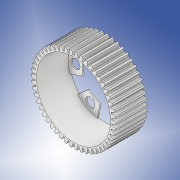
# Autodesk Inventor part: Flexspline
Saved by Autodesk Inventor 2017 SP1 (Build 210196100, 196)
## iProperties
Created: 2017-07-11
Part Number: Flexspline
Material: ABS Plastic
Document SubType Name: Modeling
Designer: zallen
Density: 1.06 g/cm^3
Appearance: CR White
Author: zallen
Autodesk Inventor part; units mm, degrees
ref_plane "YZ Plane" through (0, 0, 0) normal (1, 0, 0) x (0, 1, 0)
ref_plane "XZ Plane" through (0, 0, 0) normal (0, 1, 0) x (-1, 0, 0)
ref_plane "XY Plane" through (0, 0, 0) normal (0, 0, 1) x (1, 0, 0)
sketch "Sketch1" plane through (0, 0, 0) normal (0, 0, 1) x (1, 0, 0)
  circle A0 centre (0, 0) radius 29
  circle A1 centre (0, 0) radius 32 construction
  line L0 (0, 0) -> (52.2063, 0) construction
  arc A2 (31.9944, 0.6) -> (28.9662, 1.4) centre (26.6699, -13.4232) ccw
  arc A3 (31.9944, -0.6) -> (31.9944, 0.6) centre (12.0034, 0) ccw
  arc A4 (28.9662, -1.4) -> (31.9944, -0.6) centre (26.6699, 13.4232) ccw
  arc A5 (28.9662, -1.4) -> (28.9662, 1.4) centre (0, 0) ccw
  arc A6 (31.6669, 4.6052) -> (28.5623, 5.0194) centre (28.142, -9.9747) ccw
  arc A7 (28.9132, 2.2415) -> (31.8173, 3.4147) centre (24.7772, 16.66) ccw
  arc A8 (31.8173, 3.4147) -> (31.6669, 4.6052) centre (11.9087, 1.5044) ccw
  circle A9 centre (0, 0) radius 29
  arc A10 (28.9132, 2.2415) -> (28.5623, 5.0194) centre (0, 0) ccw
  arc A11 (30.84, 8.5378) -> (27.708, 8.5596) centre (29.1702, -6.3689) ccw
  arc A12 (28.4043, 5.8476) -> (31.1384, 7.3755) centre (22.4938, 19.634) ccw
  arc A13 (31.1384, 7.3755) -> (30.84, 8.5378) centre (11.6263, 2.9851) ccw
  circle A14 centre (0, 0) radius 29
  arc A15 (28.4043, 5.8476) -> (27.708, 8.5596) centre (0, 0) ccw
  arc A16 (29.5267, 12.3358) -> (26.4167, 11.9649) centre (29.7385, -2.6627) ccw
  arc A17 (27.4475, 9.3615) -> (29.9685, 11.22) centre (19.8556, 22.2984) ccw
  arc A18 (29.9685, 11.22) -> (29.5267, 12.3358) centre (11.1605, 4.4187) ccw
  circle A19 centre (0, 0) radius 29
  arc A20 (27.4475, 9.3615) -> (26.4167, 11.9649) centre (0, 0) ccw
  arc A21 (27.7478, 15.9392) -> (24.7088, 15.1814) centre (29.8377, 1.0855) ccw
  arc A22 (26.0577, 12.7277) -> (28.3259, 14.8876) centre (16.9043, 24.6112) ccw
  arc A23 (28.3259, 14.8876) -> (27.7478, 15.9392) centre (10.5186, 5.7827) ccw
  circle A24 centre (0, 0) radius 29
  arc A25 (26.0577, 12.7277) -> (24.7088, 15.1814) centre (0, 0) ccw
  arc A26 (25.5313, 19.2912) -> (22.6112, 18.1585) centre (29.4664, 4.8166) ccw
  arc A27 (24.257, 15.8933) -> (26.2367, 18.3204) centre (13.6864, 26.5358) ccw
  arc A28 (26.2367, 18.3204) -> (25.5313, 19.2912) centre (9.7109, 7.0554) ccw
  circle A29 centre (0, 0) radius 29
  arc A30 (24.257, 15.8933) -> (22.6112, 18.1585) centre (0, 0) ccw
  arc A31 (22.9122, 22.339) -> (20.1571, 20.8493) centre (28.6303, 8.4717) ccw
  arc A32 (22.0738, 18.8082) -> (23.7336, 21.4643) centre (10.2527, 28.0419) ccw
  arc A33 (23.7336, 21.4643) -> (22.9122, 22.339) centre (8.7501, 8.2169) ccw
  circle A34 centre (0, 0) radius 29
  arc A35 (22.0738, 18.8082) -> (20.1571, 20.8493) centre (0, 0) ccw
  arc A36 (19.9317, 25.0345) -> (17.385, 23.2112) centre (27.3428, 11.9932) ccw
  arc A37 (19.5425, 21.4264) -> (20.8563, 24.2696) centre (6.6573, 29.1058) ccw
  arc A38 (20.8563, 24.2696) -> (19.9317, 25.0345) centre (7.6512, 9.2488) ccw
  circle A39 centre (0, 0) radius 29
  arc A40 (19.5425, 21.4264) -> (17.385, 23.2112) centre (0, 0) ccw
  arc A41 (16.6368, 27.3352) -> (14.3388, 25.2071) centre (25.624, 15.3256) ccw
  arc A42 (16.7029, 23.7068) -> (17.65, 26.6922) centre (2.9569, 29.7106) ccw
  arc A43 (17.65, 26.6922) -> (16.6368, 27.3352) centre (6.4317, 10.1348) ccw
  circle A44 centre (0, 0) radius 29
  arc A45 (16.7029, 23.7068) -> (14.3388, 25.2071) centre (0, 0) ccw
  arc A46 (13.0796, 29.2048) -> (11.0664, 26.8055) centre (23.5012, 18.4163) ccw
  arc A47 (13.6, 25.6133) -> (14.1654, 28.6939) centre (-0.7902, 29.847) ccw
  arc A48 (14.1654, 28.6939) -> (13.0796, 29.2048) centre (5.1108, 10.861) ccw
  circle A49 centre (0, 0) radius 29
  arc A50 (13.6, 25.6133) -> (11.0664, 26.8055) centre (0, 0) ccw
  arc A51 (9.3162, 30.6139) -> (7.6196, 27.9811) centre (21.0077, 21.2166) ccw
  arc A52 (10.2825, 27.1159) -> (10.4574, 30.243) centre (-4.5248, 29.5126) ccw
  arc A53 (10.4574, 30.243) -> (9.3162, 30.6139) centre (3.7092, 11.4159) ccw
  circle A54 centre (0, 0) radius 29
  arc A55 (10.2825, 27.1159) -> (7.6196, 27.9811) centre (0, 0) ccw
  arc A56 (5.4058, 31.5401) -> (4.0525, 28.7155) centre (18.1829, 23.6822) ccw
  arc A57 (6.8029, 28.1908) -> (6.5845, 31.3152) centre (-8.188, 28.7128) ccw
  arc A58 (6.5845, 31.3152) -> (5.4058, 31.5401) centre (2.2492, 11.7908) ccw
  circle A59 centre (0, 0) radius 29
  arc A60 (6.8029, 28.1908) -> (4.0525, 28.7155) centre (0, 0) ccw
  arc A61 (1.4101, 31.9689) -> (0.4216, 28.9969) centre (15.0713, 25.7744) ccw
  arc A62 (3.216, 28.8211) -> (2.6078, 31.8936) centre (-11.7221, 27.4601) ccw
  arc A63 (2.6078, 31.8936) -> (1.4101, 31.9689) centre (0.7537, 11.9797) ccw
  circle A64 centre (0, 0) radius 29
  arc A65 (3.216, 28.8211) -> (0.4216, 28.9969) centre (0, 0) ccw
  arc A66 (-2.6078, 31.8936) -> (-3.216, 28.8211) centre (11.7221, 27.4601) ccw
  arc A67 (-0.4216, 28.9969) -> (-1.4101, 31.9689) centre (-15.0713, 25.7744) ccw
  arc A68 (-1.4101, 31.9689) -> (-2.6078, 31.8936) centre (-0.7537, 11.9797) ccw
  circle A69 centre (0, 0) radius 29
  arc A70 (-0.4216, 28.9969) -> (-3.216, 28.8211) centre (0, 0) ccw
  arc A71 (-6.5845, 31.3152) -> (-6.8029, 28.1908) centre (8.188, 28.7128) ccw
  arc A72 (-4.0525, 28.7155) -> (-5.4058, 31.5401) centre (-18.1829, 23.6822) ccw
  arc A73 (-5.4058, 31.5401) -> (-6.5845, 31.3152) centre (-2.2492, 11.7908) ccw
  circle A74 centre (0, 0) radius 29
  arc A75 (-4.0525, 28.7155) -> (-6.8029, 28.1908) centre (0, 0) ccw
  arc A76 (-10.4574, 30.243) -> (-10.2825, 27.1159) centre (4.5248, 29.5126) ccw
  arc A77 (-7.6196, 27.9811) -> (-9.3162, 30.6139) centre (-21.0077, 21.2166) ccw
  arc A78 (-9.3162, 30.6139) -> (-10.4574, 30.243) centre (-3.7092, 11.4159) ccw
  circle A79 centre (0, 0) radius 29
  arc A80 (-7.6196, 27.9811) -> (-10.2825, 27.1159) centre (0, 0) ccw
  arc A81 (-14.1654, 28.6939) -> (-13.6, 25.6133) centre (0.7902, 29.847) ccw
  arc A82 (-11.0664, 26.8055) -> (-13.0796, 29.2048) centre (-23.5012, 18.4163) ccw
  arc A83 (-13.0796, 29.2048) -> (-14.1654, 28.6939) centre (-5.1108, 10.861) ccw
  circle A84 centre (0, 0) radius 29
  arc A85 (-11.0664, 26.8055) -> (-13.6, 25.6133) centre (0, 0) ccw
  arc A86 (-17.65, 26.6922) -> (-16.7029, 23.7068) centre (-2.9569, 29.7106) ccw
  arc A87 (-14.3388, 25.2071) -> (-16.6368, 27.3352) centre (-25.624, 15.3256) ccw
  arc A88 (-16.6368, 27.3352) -> (-17.65, 26.6922) centre (-6.4317, 10.1348) ccw
  circle A89 centre (0, 0) radius 29
  arc A90 (-14.3388, 25.2071) -> (-16.7029, 23.7068) centre (0, 0) ccw
  arc A91 (-20.8563, 24.2696) -> (-19.5425, 21.4264) centre (-6.6573, 29.1058) ccw
  arc A92 (-17.385, 23.2112) -> (-19.9317, 25.0345) centre (-27.3428, 11.9932) ccw
  arc A93 (-19.9317, 25.0345) -> (-20.8563, 24.2696) centre (-7.6512, 9.2488) ccw
  circle A94 centre (0, 0) radius 29
  arc A95 (-17.385, 23.2112) -> (-19.5425, 21.4264) centre (0, 0) ccw
  arc A96 (-23.7336, 21.4643) -> (-22.0738, 18.8082) centre (-10.2527, 28.0419) ccw
  arc A97 (-20.1571, 20.8493) -> (-22.9122, 22.339) centre (-28.6303, 8.4717) ccw
  arc A98 (-22.9122, 22.339) -> (-23.7336, 21.4643) centre (-8.7501, 8.2169) ccw
  circle A99 centre (0, 0) radius 29
  arc A100 (-20.1571, 20.8493) -> (-22.0738, 18.8082) centre (0, 0) ccw
  arc A101 (-26.2367, 18.3204) -> (-24.257, 15.8933) centre (-13.6864, 26.5358) ccw
  arc A102 (-22.6112, 18.1585) -> (-25.5313, 19.2912) centre (-29.4664, 4.8166) ccw
  arc A103 (-25.5313, 19.2912) -> (-26.2367, 18.3204) centre (-9.7109, 7.0554) ccw
  circle A104 centre (0, 0) radius 29
  arc A105 (-22.6112, 18.1585) -> (-24.257, 15.8933) centre (0, 0) ccw
  arc A106 (-28.3259, 14.8876) -> (-26.0577, 12.7277) centre (-16.9043, 24.6112) ccw
  arc A107 (-24.7088, 15.1814) -> (-27.7478, 15.9392) centre (-29.8377, 1.0855) ccw
  arc A108 (-27.7478, 15.9392) -> (-28.3259, 14.8876) centre (-10.5186, 5.7827) ccw
  circle A109 centre (0, 0) radius 29
  arc A110 (-24.7088, 15.1814) -> (-26.0577, 12.7277) centre (0, 0) ccw
  arc A111 (-29.9685, 11.22) -> (-27.4475, 9.3615) centre (-19.8556, 22.2984) ccw
  arc A112 (-26.4167, 11.9649) -> (-29.5267, 12.3358) centre (-29.7385, -2.6627) ccw
  arc A113 (-29.5267, 12.3358) -> (-29.9685, 11.22) centre (-11.1605, 4.4187) ccw
  circle A114 centre (0, 0) radius 29
  arc A115 (-26.4167, 11.9649) -> (-27.4475, 9.3615) centre (0, 0) ccw
  arc A116 (-31.1384, 7.3755) -> (-28.4043, 5.8476) centre (-22.4938, 19.634) ccw
  arc A117 (-27.708, 8.5596) -> (-30.84, 8.5378) centre (-29.1702, -6.3689) ccw
  arc A118 (-30.84, 8.5378) -> (-31.1384, 7.3755) centre (-11.6263, 2.9851) ccw
  circle A119 centre (0, 0) radius 29
  arc A120 (-27.708, 8.5596) -> (-28.4043, 5.8476) centre (0, 0) ccw
  arc A121 (-31.8173, 3.4147) -> (-28.9132, 2.2415) centre (-24.7772, 16.66) ccw
  arc A122 (-28.5623, 5.0194) -> (-31.6669, 4.6052) centre (-28.142, -9.9747) ccw
  arc A123 (-31.6669, 4.6052) -> (-31.8173, 3.4147) centre (-11.9087, 1.5044) ccw
  circle A124 centre (0, 0) radius 29
  arc A125 (-28.5623, 5.0194) -> (-28.9132, 2.2415) centre (0, 0) ccw
  arc A126 (-31.9944, -0.6) -> (-28.9662, -1.4) centre (-26.6699, 13.4232) ccw
  arc A127 (-28.9662, 1.4) -> (-31.9944, 0.6) centre (-26.6699, -13.4232) ccw
  arc A128 (-31.9944, 0.6) -> (-31.9944, -0.6) centre (-12.0034, 0) ccw
  circle A129 centre (0, 0) radius 29
  arc A130 (-28.9662, 1.4) -> (-28.9662, -1.4) centre (0, 0) ccw
  arc A131 (-31.6669, -4.6052) -> (-28.5623, -5.0194) centre (-28.142, 9.9747) ccw
  arc A132 (-28.9132, -2.2415) -> (-31.8173, -3.4147) centre (-24.7772, -16.66) ccw
  arc A133 (-31.8173, -3.4147) -> (-31.6669, -4.6052) centre (-11.9087, -1.5044) ccw
  circle A134 centre (0, 0) radius 29
  arc A135 (-28.9132, -2.2415) -> (-28.5623, -5.0194) centre (0, 0) ccw
  arc A136 (-30.84, -8.5378) -> (-27.708, -8.5596) centre (-29.1702, 6.3689) ccw
  arc A137 (-28.4043, -5.8476) -> (-31.1384, -7.3755) centre (-22.4938, -19.634) ccw
  arc A138 (-31.1384, -7.3755) -> (-30.84, -8.5378) centre (-11.6263, -2.9851) ccw
  circle A139 centre (0, 0) radius 29
  arc A140 (-28.4043, -5.8476) -> (-27.708, -8.5596) centre (0, 0) ccw
  arc A141 (-29.5267, -12.3358) -> (-26.4167, -11.9649) centre (-29.7385, 2.6627) ccw
  arc A142 (-27.4475, -9.3615) -> (-29.9685, -11.22) centre (-19.8556, -22.2984) ccw
  arc A143 (-29.9685, -11.22) -> (-29.5267, -12.3358) centre (-11.1605, -4.4187) ccw
  circle A144 centre (0, 0) radius 29
  arc A145 (-27.4475, -9.3615) -> (-26.4167, -11.9649) centre (0, 0) ccw
  arc A146 (-27.7478, -15.9392) -> (-24.7088, -15.1814) centre (-29.8377, -1.0855) ccw
  arc A147 (-26.0577, -12.7277) -> (-28.3259, -14.8876) centre (-16.9043, -24.6112) ccw
  arc A148 (-28.3259, -14.8876) -> (-27.7478, -15.9392) centre (-10.5186, -5.7827) ccw
  circle A149 centre (0, 0) radius 29
  arc A150 (-26.0577, -12.7277) -> (-24.7088, -15.1814) centre (0, 0) ccw
  arc A151 (-25.5313, -19.2912) -> (-22.6112, -18.1585) centre (-29.4664, -4.8166) ccw
  arc A152 (-24.257, -15.8933) -> (-26.2367, -18.3204) centre (-13.6864, -26.5358) ccw
  arc A153 (-26.2367, -18.3204) -> (-25.5313, -19.2912) centre (-9.7109, -7.0554) ccw
  circle A154 centre (0, 0) radius 29
  arc A155 (-24.257, -15.8933) -> (-22.6112, -18.1585) centre (0, 0) ccw
  arc A156 (-22.9122, -22.339) -> (-20.1571, -20.8493) centre (-28.6303, -8.4717) ccw
  arc A157 (-22.0738, -18.8082) -> (-23.7336, -21.4643) centre (-10.2527, -28.0419) ccw
  arc A158 (-23.7336, -21.4643) -> (-22.9122, -22.339) centre (-8.7501, -8.2169) ccw
  circle A159 centre (0, 0) radius 29
  arc A160 (-22.0738, -18.8082) -> (-20.1571, -20.8493) centre (0, 0) ccw
  arc A161 (-19.9317, -25.0345) -> (-17.385, -23.2112) centre (-27.3428, -11.9932) ccw
  arc A162 (-19.5425, -21.4264) -> (-20.8563, -24.2696) centre (-6.6573, -29.1058) ccw
  arc A163 (-20.8563, -24.2696) -> (-19.9317, -25.0345) centre (-7.6512, -9.2488) ccw
  circle A164 centre (0, 0) radius 29
  arc A165 (-19.5425, -21.4264) -> (-17.385, -23.2112) centre (0, 0) ccw
  arc A166 (-16.6368, -27.3352) -> (-14.3388, -25.2071) centre (-25.624, -15.3256) ccw
  arc A167 (-16.7029, -23.7068) -> (-17.65, -26.6922) centre (-2.9569, -29.7106) ccw
  arc A168 (-17.65, -26.6922) -> (-16.6368, -27.3352) centre (-6.4317, -10.1348) ccw
  circle A169 centre (0, 0) radius 29
  arc A170 (-16.7029, -23.7068) -> (-14.3388, -25.2071) centre (0, 0) ccw
  arc A171 (-13.0796, -29.2048) -> (-11.0664, -26.8055) centre (-23.5012, -18.4163) ccw
  arc A172 (-13.6, -25.6133) -> (-14.1654, -28.6939) centre (0.7902, -29.847) ccw
  arc A173 (-14.1654, -28.6939) -> (-13.0796, -29.2048) centre (-5.1108, -10.861) ccw
  circle A174 centre (0, 0) radius 29
  arc A175 (-13.6, -25.6133) -> (-11.0664, -26.8055) centre (0, 0) ccw
  arc A176 (-9.3162, -30.6139) -> (-7.6196, -27.9811) centre (-21.0077, -21.2166) ccw
  arc A177 (-10.2825, -27.1159) -> (-10.4574, -30.243) centre (4.5248, -29.5126) ccw
  arc A178 (-10.4574, -30.243) -> (-9.3162, -30.6139) centre (-3.7092, -11.4159) ccw
  circle A179 centre (0, 0) radius 29
  arc A180 (-10.2825, -27.1159) -> (-7.6196, -27.9811) centre (0, 0) ccw
  arc A181 (-5.4058, -31.5401) -> (-4.0525, -28.7155) centre (-18.1829, -23.6822) ccw
  arc A182 (-6.8029, -28.1908) -> (-6.5845, -31.3152) centre (8.188, -28.7128) ccw
  arc A183 (-6.5845, -31.3152) -> (-5.4058, -31.5401) centre (-2.2492, -11.7908) ccw
  circle A184 centre (0, 0) radius 29
  arc A185 (-6.8029, -28.1908) -> (-4.0525, -28.7155) centre (0, 0) ccw
  arc A186 (-1.4101, -31.9689) -> (-0.4216, -28.9969) centre (-15.0713, -25.7744) ccw
  arc A187 (-3.216, -28.8211) -> (-2.6078, -31.8936) centre (11.7221, -27.4601) ccw
  arc A188 (-2.6078, -31.8936) -> (-1.4101, -31.9689) centre (-0.7537, -11.9797) ccw
  circle A189 centre (0, 0) radius 29
  arc A190 (-3.216, -28.8211) -> (-0.4216, -28.9969) centre (0, 0) ccw
  arc A191 (2.6078, -31.8936) -> (3.216, -28.8211) centre (-11.7221, -27.4601) ccw
  arc A192 (0.4216, -28.9969) -> (1.4101, -31.9689) centre (15.0713, -25.7744) ccw
  arc A193 (1.4101, -31.9689) -> (2.6078, -31.8936) centre (0.7537, -11.9797) ccw
  circle A194 centre (0, 0) radius 29
  arc A195 (0.4216, -28.9969) -> (3.216, -28.8211) centre (0, 0) ccw
  arc A196 (6.5845, -31.3152) -> (6.8029, -28.1908) centre (-8.188, -28.7128) ccw
  arc A197 (4.0525, -28.7155) -> (5.4058, -31.5401) centre (18.1829, -23.6822) ccw
  arc A198 (5.4058, -31.5401) -> (6.5845, -31.3152) centre (2.2492, -11.7908) ccw
  circle A199 centre (0, 0) radius 29
  arc A200 (4.0525, -28.7155) -> (6.8029, -28.1908) centre (0, 0) ccw
  arc A201 (10.4574, -30.243) -> (10.2825, -27.1159) centre (-4.5248, -29.5126) ccw
  arc A202 (7.6196, -27.9811) -> (9.3162, -30.6139) centre (21.0077, -21.2166) ccw
  arc A203 (9.3162, -30.6139) -> (10.4574, -30.243) centre (3.7092, -11.4159) ccw
  circle A204 centre (0, 0) radius 29
  arc A205 (7.6196, -27.9811) -> (10.2825, -27.1159) centre (0, 0) ccw
  arc A206 (14.1654, -28.6939) -> (13.6, -25.6133) centre (-0.7902, -29.847) ccw
  arc A207 (11.0664, -26.8055) -> (13.0796, -29.2048) centre (23.5012, -18.4163) ccw
  arc A208 (13.0796, -29.2048) -> (14.1654, -28.6939) centre (5.1108, -10.861) ccw
  circle A209 centre (0, 0) radius 29
  arc A210 (11.0664, -26.8055) -> (13.6, -25.6133) centre (0, 0) ccw
  arc A211 (17.65, -26.6922) -> (16.7029, -23.7068) centre (2.9569, -29.7106) ccw
  arc A212 (14.3388, -25.2071) -> (16.6368, -27.3352) centre (25.624, -15.3256) ccw
  arc A213 (16.6368, -27.3352) -> (17.65, -26.6922) centre (6.4317, -10.1348) ccw
  circle A214 centre (0, 0) radius 29
  arc A215 (14.3388, -25.2071) -> (16.7029, -23.7068) centre (0, 0) ccw
  arc A216 (20.8563, -24.2696) -> (19.5425, -21.4264) centre (6.6573, -29.1058) ccw
  arc A217 (17.385, -23.2112) -> (19.9317, -25.0345) centre (27.3428, -11.9932) ccw
  arc A218 (19.9317, -25.0345) -> (20.8563, -24.2696) centre (7.6512, -9.2488) ccw
  circle A219 centre (0, 0) radius 29
  arc A220 (17.385, -23.2112) -> (19.5425, -21.4264) centre (0, 0) ccw
  arc A221 (23.7336, -21.4643) -> (22.0738, -18.8082) centre (10.2527, -28.0419) ccw
  arc A222 (20.1571, -20.8493) -> (22.9122, -22.339) centre (28.6303, -8.4717) ccw
  arc A223 (22.9122, -22.339) -> (23.7336, -21.4643) centre (8.7501, -8.2169) ccw
  circle A224 centre (0, 0) radius 29
  arc A225 (20.1571, -20.8493) -> (22.0738, -18.8082) centre (0, 0) ccw
  arc A226 (26.2367, -18.3204) -> (24.257, -15.8933) centre (13.6864, -26.5358) ccw
  arc A227 (22.6112, -18.1585) -> (25.5313, -19.2912) centre (29.4664, -4.8166) ccw
  arc A228 (25.5313, -19.2912) -> (26.2367, -18.3204) centre (9.7109, -7.0554) ccw
  circle A229 centre (0, 0) radius 29
  arc A230 (22.6112, -18.1585) -> (24.257, -15.8933) centre (0, 0) ccw
  arc A231 (28.3259, -14.8876) -> (26.0577, -12.7277) centre (16.9043, -24.6112) ccw
  arc A232 (24.7088, -15.1814) -> (27.7478, -15.9392) centre (29.8377, -1.0855) ccw
  arc A233 (27.7478, -15.9392) -> (28.3259, -14.8876) centre (10.5186, -5.7827) ccw
  circle A234 centre (0, 0) radius 29
  arc A235 (24.7088, -15.1814) -> (26.0577, -12.7277) centre (0, 0) ccw
  arc A236 (29.9685, -11.22) -> (27.4475, -9.3615) centre (19.8556, -22.2984) ccw
  arc A237 (26.4167, -11.9649) -> (29.5267, -12.3358) centre (29.7385, 2.6627) ccw
  arc A238 (29.5267, -12.3358) -> (29.9685, -11.22) centre (11.1605, -4.4187) ccw
  circle A239 centre (0, 0) radius 29
  arc A240 (26.4167, -11.9649) -> (27.4475, -9.3615) centre (0, 0) ccw
  arc A241 (31.1384, -7.3755) -> (28.4043, -5.8476) centre (22.4938, -19.634) ccw
  arc A242 (27.708, -8.5596) -> (30.84, -8.5378) centre (29.1702, 6.3689) ccw
  arc A243 (30.84, -8.5378) -> (31.1384, -7.3755) centre (11.6263, -2.9851) ccw
  circle A244 centre (0, 0) radius 29
  arc A245 (27.708, -8.5596) -> (28.4043, -5.8476) centre (0, 0) ccw
  arc A246 (31.8173, -3.4147) -> (28.9132, -2.2415) centre (24.7772, -16.66) ccw
  arc A247 (28.5623, -5.0194) -> (31.6669, -4.6052) centre (28.142, 9.9747) ccw
  arc A248 (31.6669, -4.6052) -> (31.8173, -3.4147) centre (11.9087, -1.5044) ccw
  circle A249 centre (0, 0) radius 29
  arc A250 (28.5623, -5.0194) -> (28.9132, -2.2415) centre (0, 0) ccw
  point P0 (32.0034, 0)
  point P1 (31.751, 4.0111)
  point P2 (30.9979, 7.9589)
  point P3 (29.756, 11.7812)
  point P4 (28.0448, 15.4177)
  point P5 (25.8913, 18.8111)
  point P6 (23.3295, 21.9078)
  point P7 (20.3997, 24.659)
  point P8 (17.1483, 27.0213)
  point P9 (13.6264, 28.9575)
  point P10 (9.8896, 30.437)
  point P11 (5.9968, 31.4365)
  point P12 (2.0095, 31.9402)
  point P13 (-2.0095, 31.9402)
  point P14 (-5.9968, 31.4365)
  point P15 (-9.8896, 30.437)
  point P16 (-13.6264, 28.9575)
  point P17 (-17.1483, 27.0213)
  point P18 (-20.3997, 24.659)
  point P19 (-23.3295, 21.9078)
  point P20 (-25.8913, 18.8111)
  point P21 (-28.0448, 15.4177)
  point P22 (-29.756, 11.7812)
  point P23 (-30.9979, 7.9589)
  point P24 (-31.751, 4.0111)
  point P25 (-32.0034, 0)
  point P26 (-31.751, -4.0111)
  point P27 (-30.9979, -7.9589)
  point P28 (-29.756, -11.7812)
  point P29 (-28.0448, -15.4177)
  point P30 (-25.8913, -18.8111)
  point P31 (-23.3295, -21.9078)
  point P32 (-20.3997, -24.659)
  point P33 (-17.1483, -27.0213)
  point P34 (-13.6264, -28.9575)
  point P35 (-9.8896, -30.437)
  point P36 (-5.9968, -31.4365)
  point P37 (-2.0095, -31.9402)
  point P38 (2.0095, -31.9402)
  point P39 (5.9968, -31.4365)
  point P40 (9.8896, -30.437)
  point P41 (13.6264, -28.9575)
  point P42 (17.1483, -27.0213)
  point P43 (20.3997, -24.659)
  point P44 (23.3295, -21.9078)
  point P45 (25.8913, -18.8111)
  point P46 (28.0448, -15.4177)
  point P47 (29.756, -11.7812)
  point P48 (30.9979, -7.9589)
  point P49 (31.751, -4.0111)
  dimension "d0" = 58
  dimension "d2" = 15
  dimension "d3" = 20
  dimension "d4" = 1.2
  dimension "d5" = 1.4
  dimension "d6" = 3
  dimension "d9" = 360
  constraints: 403 point on circle, 201 centre point, 2 coincident, 2 end point, 2 symmetric about line, 1 horizontal, 1 point on line, 952 other
  measures "d2" radius of A2
  measures "d3" radius of A3
  measures "d4" distance of A1.end A1.start
  measures "d5" distance from line of L0 A2.end
extrude "Extrusion1" add sketch "Sketch1" along normal blind 24
sketch "Sketch2" plane through (0, 0, 24) normal (0, 0, 1) x (1, 0, 0)
  circle A0 centre (0, 0) radius 28
  dimension "d13" = 56
  constraints: 1 centre point, 1 coincident
  measures "d13" diameter of A0
extrude "Extrusion2" cut sketch "Sketch2" against normal through all
sketch "Sketch3" plane through (0, 0, 0) normal (0, 0, -1) x (-1, 0, 0)
  circle A0 centre (0, 0) radius 11
  circle A1 centre (0, 0) radius 17.5 construction
  circle A2 centre (0, 0) radius 28 construction
  line L0 (-6, 27.3496) -> (-4, 17.0367)
  line L1 (6, 27.3496) -> (4, 17.0367)
  arc A3 (6, 27.3496) -> (-6, 27.3496) centre (0, 0) ccw
  arc A4 (4, 17.0367) -> (-4, 17.0367) centre (0, 0) ccw
  circle A5 centre (0, 0) radius 22.5 construction
  line L2 (4.9525, 21.9482) -> (16.5314, 15.2631) construction
  line L3 (10.742, 18.6056) -> (11.25, 19.4856) construction
  circle A6 centre (11.25, 19.4856) radius 3.5
  circle A7 centre (-11.25, 19.4856) radius 3.5
  circle A8 centre (-22.5, 0) radius 3.5
  circle A9 centre (-11.25, -19.4856) radius 3.5
  circle A10 centre (11.25, -19.4856) radius 3.5
  circle A11 centre (22.5, 0) radius 3.5
  arc A12 (-20.6854, 18.8709) -> (-26.6854, 8.4786) centre (0, 0) ccw
  line L4 (-20.6854, 18.8709) -> (-12.7542, 11.9825)
  line L5 (-26.6854, 8.4786) -> (-16.7542, 5.0543)
  arc A13 (-12.7542, 11.9825) -> (-16.7542, 5.0543) centre (0, 0) ccw
  arc A14 (-26.6854, -8.4786) -> (-20.6854, -18.8709) centre (0, 0) ccw
  line L6 (-26.6854, -8.4786) -> (-16.7542, -5.0543)
  line L7 (-20.6854, -18.8709) -> (-12.7542, -11.9825)
  arc A15 (-16.7542, -5.0543) -> (-12.7542, -11.9825) centre (0, 0) ccw
  arc A16 (-6, -27.3496) -> (6, -27.3496) centre (0, 0) ccw
  line L8 (-6, -27.3496) -> (-4, -17.0367)
  line L9 (6, -27.3496) -> (4, -17.0367)
  arc A17 (-4, -17.0367) -> (4, -17.0367) centre (0, 0) ccw
  arc A18 (20.6854, -18.8709) -> (26.6854, -8.4786) centre (0, 0) ccw
  line L10 (20.6854, -18.8709) -> (12.7542, -11.9825)
  line L11 (26.6854, -8.4786) -> (16.7542, -5.0543)
  arc A19 (12.7542, -11.9825) -> (16.7542, -5.0543) centre (0, 0) ccw
  arc A20 (26.6854, 8.4786) -> (20.6854, 18.8709) centre (0, 0) ccw
  line L12 (26.6854, 8.4786) -> (16.7542, 5.0543)
  line L13 (20.6854, 18.8709) -> (12.7542, 11.9825)
  arc A21 (16.7542, 5.0543) -> (12.7542, 11.9825) centre (0, 0) ccw
  circle A22 centre (0, 0) radius 29
  point P0 (-16.5314, 15.2631)
  point P1 (-21.4839, -6.6851)
  point P2 (-4.9525, -21.9482)
  point P3 (16.5314, -15.2631)
  point P4 (21.4839, 6.6851)
  dimension "d16" = 22
  dimension "d17" = 35
  dimension "d18" = 56
  dimension "d20" = 6
  dimension "d21" = 4
  dimension "d22" = 6
  dimension "d23" = 4
  dimension "d28" = 45
  dimension "d29" = 7
  dimension "d32" = 360
  dimension "d38" = 360
  dimension "d44" = 58
  constraints: 31 point on circle, 28 end point, 23 centre point, 7 point on line, 5 coincident, 3 concentric, 1 midpoint, 1 perpendicular, 80 other
  measures "d16" diameter of A0
  measures "d17" diameter of A1
  measures "d18" diameter of A2
  measures "d20" horizontal distance of point (0, 0) L0.start
  measures "d21" horizontal distance of point (0, 0) L0.end
  measures "d22" horizontal distance of point (0, 0) L1.start
  measures "d23" horizontal distance of point (0, 0) L1.end
  measures "d28" diameter of A5
  measures "d29" diameter of A6
  measures "d44" diameter of A22
extrude "Extrusion4" add sketch "Sketch3" along normal blind 1
sketch "Sketch4" plane through (0, 0, -1) normal (0, 0, -1) x (-1, 0, 0)
  circle A0 centre (0, 0) radius 17.5
  arc A1 (-12.0237, 12.7154) -> (-17.0237, 4.0551) centre (0, 0) ccw
  line L0 (0, 0) -> (-15.1554, 8.75) construction
  arc A2 (-12.0237, 12.7154) -> (-17.0237, 4.0551) centre (0, 0) ccw
  constraints: 7 point on circle, 2 centre point, 2 end point, 1 coincident, 4 other
extrude "Extrusion5" cut sketch "Sketch4" against normal through all
body "Solid1"
